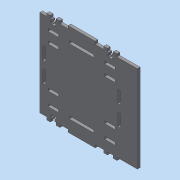
# Autodesk Inventor part: Base
Saved by Autodesk Inventor 2016 SP1 (Build 200210100, 210)
## iProperties
Created: 2016-03-01
Part Number: Base
Material: Generic
Document SubType Name: Modeling
Designer: Mohamed A.
Density: 1 g/cm^3
Appearance: Default
Author: Mohamed A.
Autodesk Inventor part; units mm, degrees
note: some values were not read from the file. Chosen so that the rebuilt part matches the saved one: sketch regions of "Extrusion1".
ref_plane "YZ Plane" through (0, 0, 0) normal (1, 0, 0) x (0, 1, 0)
ref_plane "XZ Plane" through (0, 0, 0) normal (0, 1, 0) x (-1, 0, 0)
ref_plane "XY Plane" through (0, 0, 0) normal (0, 0, 1) x (1, 0, 0)
sketch "Sketch2" plane through (0, 0, 0) normal (0, 1, 0) x (-1, 0, 0)
  line L0 (53.75, 51) -> (46.25, 51)
  line L1 (-53.75, 51) -> (-53.75, 48)
  line L2 (-53.75, -51) -> (-31.25, -51)
  line L3 (53.75, 51) -> (53.75, -51)
  line L4 (75.25, 0) -> (-75.25, 0) construction
  line L5 (0, -71.4) -> (0, 71.4) construction
  line L6 (-53.75, -48) -> (-31.25, -48)
  line L7 (46.25, -48) -> (46.25, -51)
  line L8 (31.75, -48) -> (31.75, -51)
  line L9 (22.75, -48) -> (22.75, -51)
  line L10 (-7.25, -48) -> (-7.25, -51)
  line L11 (46.25, -51) -> (53.75, -51)
  line L12 (31.75, -51) -> (46.25, -51)
  line L13 (22.75, -51) -> (31.75, -51)
  line L14 (-7.25, -51) -> (22.75, -51)
  line L15 (-17.75, -51) -> (-16.75, -51)
  line L16 (-53.75, -48) -> (-31.25, -48)
  line L17 (22.75, -48) -> (31.75, -48)
  line L18 (31.75, -48) -> (37.5, -48)
  line L19 (46.25, -48) -> (53.75, -48)
  line L20 (39, -51) -> (39, -34.4895) construction
  line L21 (37.5, -48) -> (37.5, -46)
  line L22 (37.5, -46) -> (36.35, -46)
  line L23 (36.35, -46) -> (36.35, -43.6)
  line L24 (36.35, -43.6) -> (37.5, -43.6)
  line L25 (37.5, -43.6) -> (37.5, -43)
  line L26 (37.5, -43) -> (40.5, -43)
  line L27 (40.5, -43) -> (40.5, -43.6)
  line L28 (40.5, -43.6) -> (41.65, -43.6)
  line L29 (41.65, -43.6) -> (41.65, -46)
  line L30 (41.65, -46) -> (40.5, -46)
  line L31 (40.5, -48) -> (40.5, -46)
  line L32 (37.5, -48) -> (40.5, -48)
  line L33 (40.5, -48) -> (46.25, -48)
  line L34 (35.75, -48) -> (35.75, -51)
  line L35 (42.25, -51) -> (42.25, -48)
  line L36 (-53.75, -48) -> (-53.75, -51)
  line L37 (-53.75, 48) -> (-53.75, -48)
  line L38 (-24, -51) -> (-24, -36.3638) construction
  line L39 (-25.5, -48) -> (-25.5, -46)
  line L40 (-25.5, -46) -> (-26.65, -46)
  line L41 (-26.65, -46) -> (-26.65, -43.6)
  line L42 (-26.65, -43.6) -> (-25.5, -43.6)
  line L43 (-25.5, -43.6) -> (-25.5, -43)
  line L44 (-25.5, -43) -> (-22.5, -43)
  line L45 (-22.5, -43) -> (-22.5, -43.6)
  line L46 (-22.5, -43.6) -> (-21.35, -43.6)
  line L47 (-21.35, -43.6) -> (-21.35, -46)
  line L48 (-21.35, -46) -> (-22.5, -46)
  line L49 (-22.5, -46) -> (-22.5, -48)
  line L50 (-20.75, -51) -> (-20.75, -48)
  line L51 (-16.75, -51) -> (-16.75, -48)
  line L52 (-27.25, -48) -> (-27.25, -51)
  line L53 (-31.25, -48) -> (-31.25, -51)
  line L54 (-27.25, -48) -> (22.75, -48)
  line L55 (-25.5, -48) -> (-22.5, -48)
  line L56 (-31.25, -48) -> (-27.25, -48)
  line L57 (-31.25, -51) -> (-27.25, -51)
  line L58 (-27.25, -51) -> (-20.75, -51)
  line L59 (-31.25, -48) -> (-27.25, -48)
  line L60 (-16.75, -51) -> (-7.25, -51)
  line L61 (-16.75, -48) -> (-7.25, -48)
  line L62 (-27.25, -48) -> (-25.5, -48)
  line L63 (-53.75, 48) -> (-31.25, 48)
  line L64 (46.25, 48) -> (46.25, 51)
  line L65 (31.75, 48) -> (31.75, 51)
  line L66 (22.75, 48) -> (22.75, 51)
  line L67 (-7.25, 48) -> (-7.25, 51)
  line L68 (37.5, 48) -> (37.5, 46)
  line L69 (37.5, 46) -> (36.35, 46)
  line L70 (36.35, 46) -> (36.35, 43.6)
  line L71 (36.35, 43.6) -> (37.5, 43.6)
  line L72 (37.5, 43.6) -> (37.5, 43)
  line L73 (37.5, 43) -> (40.5, 43)
  line L74 (40.5, 43) -> (40.5, 43.6)
  line L75 (40.5, 43.6) -> (41.65, 43.6)
  line L76 (41.65, 43.6) -> (41.65, 46)
  line L77 (41.65, 46) -> (40.5, 46)
  line L78 (40.5, 48) -> (40.5, 46)
  line L79 (35.75, 48) -> (35.75, 51)
  line L80 (42.25, 51) -> (42.25, 48)
  line L81 (-25.5, 48) -> (-25.5, 46)
  line L82 (-25.5, 46) -> (-26.65, 46)
  line L83 (-26.65, 46) -> (-26.65, 43.6)
  line L84 (-26.65, 43.6) -> (-25.5, 43.6)
  line L85 (-25.5, 43.6) -> (-25.5, 43)
  line L86 (-25.5, 43) -> (-22.5, 43)
  line L87 (-22.5, 43) -> (-22.5, 43.6)
  line L88 (-22.5, 43.6) -> (-21.35, 43.6)
  line L89 (-21.35, 43.6) -> (-21.35, 46)
  line L90 (-21.35, 46) -> (-22.5, 46)
  line L91 (-22.5, 46) -> (-22.5, 48)
  line L92 (-20.75, 51) -> (-20.75, 48)
  line L93 (-16.75, 51) -> (-16.75, 48)
  line L94 (-27.25, 48) -> (-27.25, 51)
  line L95 (-31.25, 48) -> (-31.25, 51)
  line L96 (-31.25, 51) -> (-53.75, 51)
  line L97 (-31.25, 48) -> (-27.25, 48)
  line L98 (-27.25, 51) -> (-31.25, 51)
  line L99 (-27.25, 48) -> (-25.5, 48)
  line L100 (-25.5, 48) -> (-22.5, 48)
  line L101 (-22.5, 48) -> (-20.75, 48)
  line L102 (-20.75, 51) -> (-27.25, 51)
  line L103 (-20.75, 48) -> (-16.75, 48)
  line L104 (-16.75, 48) -> (-7.25, 48)
  line L105 (-16.75, 51) -> (-20.75, 51)
  line L106 (-7.25, 51) -> (-16.75, 51)
  line L107 (-7.25, 48) -> (22.75, 48)
  line L108 (22.75, 51) -> (-7.25, 51)
  line L109 (22.75, 48) -> (31.75, 48)
  line L110 (31.75, 51) -> (22.75, 51)
  line L111 (31.75, 48) -> (35.75, 48)
  line L112 (35.75, 51) -> (31.75, 51)
  line L113 (35.75, 48) -> (37.5, 48)
  line L114 (37.5, 48) -> (40.5, 48)
  line L115 (40.5, 48) -> (42.25, 48)
  line L116 (42.25, 48) -> (46.25, 48)
  line L117 (42.25, 51) -> (35.75, 51)
  line L118 (46.25, 51) -> (42.25, 51)
  line L119 (46.25, 48) -> (53.75, 48)
  line L120 (-32.25, 3.975) -> (-32.25, 18) projected
  line L121 (-32.25, 18) -> (-35.25, 18) projected
  line L122 (-35.25, 3.975) -> (-35.25, 18) projected
  line L123 (-32.25, 3.975) -> (-35.25, 3.975) projected
  line L124 (-32.25, -18) -> (-32.25, -3.975) projected
  line L125 (-32.25, -3.975) -> (-35.25, -3.975) projected
  line L126 (-35.25, -18) -> (-35.25, -3.975) projected
  line L127 (-32.25, -18) -> (-35.25, -18) projected
  line L128 (-29.25, 21) -> (-17.75, 21) projected
  line L129 (-17.75, 21) -> (-17.75, 24) projected
  line L130 (-29.25, 24) -> (-17.75, 24) projected
  line L131 (-29.25, 21) -> (-29.25, 24) projected
  line L132 (-17.75, 37.4948) -> (-17.75, 34.4948) projected
  line L133 (-29.25, 37.4948) -> (-17.75, 37.4948) projected
  line L134 (-29.25, 34.4948) -> (-29.25, 37.4948) projected
  line L135 (-17.75, 34.4948) -> (-29.25, 34.4948) projected
  line L136 (-29.25, -34.5052) -> (-29.25, -37.5052) projected
  line L137 (-17.75, -37.5052) -> (-29.25, -37.5052) projected
  line L138 (-17.75, -37.5052) -> (-17.75, -34.5052) projected
  line L139 (-29.25, -34.5052) -> (-17.75, -34.5052) projected
  line L140 (-29.25, -24) -> (-17.75, -24) projected
  line L141 (-17.75, -24) -> (-17.75, -21) projected
  line L142 (-29.25, -21) -> (-17.75, -21) projected
  line L143 (-29.25, -24) -> (-29.25, -21) projected
  line L144 (-5.75, -34.5052) -> (-5.75, -37.5052) projected
  line L145 (21.25, -37.5052) -> (-5.75, -37.5052) projected
  line L146 (21.25, -37.5052) -> (21.25, -34.5052) projected
  line L147 (-5.75, -34.5052) -> (21.25, -34.5052) projected
  line L148 (21.25, 34.4948) -> (21.25, 37.4948) projected
  line L149 (-5.75, 37.4948) -> (21.25, 37.4948) projected
  line L150 (-5.75, 37.4948) -> (-5.75, 34.4948) projected
  line L151 (21.25, 34.4948) -> (-5.75, 34.4948) projected
  line L152 (33.25, 21) -> (44.75, 21) projected
  line L153 (44.75, 21) -> (44.75, 24) projected
  line L154 (33.25, 24) -> (44.75, 24) projected
  line L155 (33.25, 21) -> (33.25, 24) projected
  line L156 (44.75, 34.4948) -> (44.75, 37.4948) projected
  line L157 (33.25, 37.4948) -> (44.75, 37.4948) projected
  line L158 (33.25, 37.4948) -> (33.25, 34.4948) projected
  line L159 (44.75, 34.4948) -> (33.25, 34.4948) projected
  line L160 (33.25, -37.5052) -> (33.25, -34.5052) projected
  line L161 (44.75, -37.5052) -> (33.25, -37.5052) projected
  line L162 (44.75, -34.5052) -> (44.75, -37.5052) projected
  line L163 (33.25, -34.5052) -> (44.75, -34.5052) projected
  line L164 (33.25, -24) -> (44.75, -24) projected
  line L165 (44.75, -24) -> (44.75, -21) projected
  line L166 (33.25, -21) -> (44.75, -21) projected
  line L167 (33.25, -24) -> (33.25, -21) projected
  line L168 (50.75, -18) -> (50.75, -3.975) projected
  line L169 (50.75, -3.975) -> (47.75, -3.975) projected
  line L170 (47.75, -18) -> (47.75, -3.975) projected
  line L171 (50.75, -18) -> (47.75, -18) projected
  line L172 (50.75, 3.975) -> (50.75, 18) projected
  line L173 (50.75, 18) -> (47.75, 18) projected
  line L174 (47.75, 3.975) -> (47.75, 18) projected
  line L175 (50.75, 3.975) -> (47.75, 3.975) projected
  line L176 (-32.25, 3.975) -> (-35.25, -3.975) construction
  line L177 (-32.25, -3.975) -> (-35.25, 3.975) construction
  line L178 (50.75, -3.975) -> (47.75, 3.975) construction
  line L179 (50.75, 3.975) -> (47.75, -3.975) construction
  circle A0 centre (49.25, 0) radius 1.4
  circle A1 centre (-33.75, 0) radius 1.4
  line L180 (-22.5, -48) -> (-20.75, -48)
  line L181 (-20.75, -48) -> (-16.75, -48)
  line L182 (-20.75, -51) -> (-7.25, -51)
  point P0 (0, 0)
  dimension "d1" = 102
  dimension "d5" = 107.5
  dimension "d6" = 3
  dimension "d7" = 7.5
  dimension "d8" = 14.5
  dimension "d9" = 9
  dimension "d10" = 30
  dimension "d13" = 2.4
  dimension "d14" = 5.3
  dimension "d15" = 2
  dimension "d16" = 5
  dimension "d17" = 3
  dimension "d18" = 6.5
  dimension "d24" = 6.5
  dimension "d25" = 14.5
  dimension "d26" = 9.5
  dimension "d28" = 2.8
  dimension "d29" = 2.8
  constraints: 248 end point, 145 perpendicular, 112 parallel, 47 point on line, 44 symmetric about line, 11 horizontal, 7 collinear, 6 vertical, 4 midpoint, 2 centre point, 19 other
  measures "d1" distance of L1.start L2.start
  measures "d5" distance between parallel lines of L3 L1
  measures "d6" distance between parallel lines of L2 L6
  measures "d7" distance between parallel lines of L3 L7
  measures "d8" distance between parallel lines of L7 L8
  measures "d9" distance between parallel lines of L8 L9
  measures "d10" distance between parallel lines of L10 L9
  measures "d13" distance between parallel lines of L30 L28
  measures "d14" distance between parallel lines of L29 L23
  measures "d15" distance between parallel lines of L18 L30
  measures "d16" distance between parallel lines of L18 L26
  measures "d17" distance between parallel lines of L27 L25
  measures "d18" distance between parallel lines of L35 L34
  measures "d24" distance between parallel lines of L50 L52
  measures "d25" distance between parallel lines of L51 L53
  measures "d26" distance between parallel lines of L51 L10
  measures "d28" diameter of A0
  measures "d29" diameter of A1
extrude "Extrusion1" add sketch "Sketch2" along normal blind 3 contours L64 L116 L80 L118 | L3 L19 L33 L31 L30 L29 L28 L27 L26 L25 L24 L23 L22 L21 L18 L17 L54 L49 L48 L47 L46 L45 L44 L43 L42 L41 L40 L39 L56 L6 L37 L63 L97 L99 L81 L82 L83 L84 L85 L86 L87 L88 L89 L90 L91 L101 L103 L104 L107 L109 L111 L113 L68 L69 L70 L71 L72 L73 L74 L75 L76 L77 L78 L115 L116 L119 | L79 L111 L65 L112 | L7 L12 L35 L33 | L66 L107 L67 L108 | L12 L8 L18 L34 | L93 L103 L92 L105 | L14 L10 L54 L9 | L94 L97 L95 L98 | L15 L182 L50 L54 L51 | L57 L53 L56 L52
body "Solid1"
